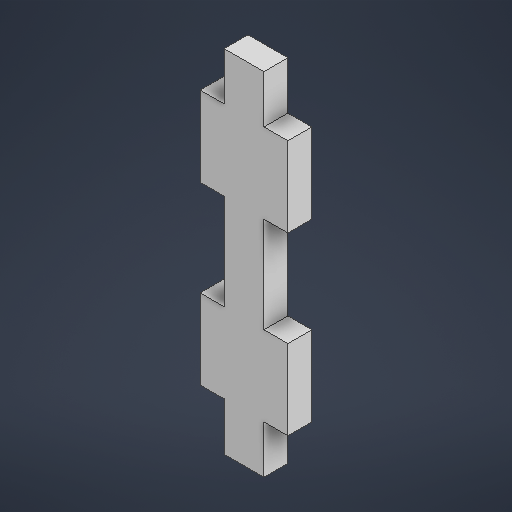
# Autodesk Inventor part: columna2
Saved by Autodesk Inventor 2026 (Build 300175000, 175)
## iProperties
Created: 2026-05-15
Part Number: columna2
Material: Generic
Document SubType Name: Modeling
Designer: juana
Density: 1 g/cm^3
Appearance: Default
Author: juana
Autodesk Inventor part; units mm, degrees
ref_plane "YZ Plane" through (0, 0, 0) normal (1, 0, 0) x (0, 1, 0)
ref_plane "XZ Plane" through (0, 0, 0) normal (0, 1, 0) x (-1, 0, 0)
ref_plane "XY Plane" through (0, 0, 0) normal (0, 0, 1) x (1, 0, 0)
sketch "Sketch1" plane through (0, 0, 0) normal (0, 0, 1) x (1, 0, 0)
  line L0 (0, 0) -> (5, 0)
  line L1 (5, 0) -> (5, 44)
  line L2 (5, 44) -> (0, 44)
  line L3 (0, 44) -> (0, 0)
  line L4 (5, 6) -> (8, 6)
  line L5 (8, 6) -> (8, 16)
  line L6 (8, 16) -> (5, 16)
  line L7 (5, 16) -> (5, 6)
  line L8 (5, 22) -> (0, 22) construction
  line L9 (2.5, 22) -> (2.5, 0) construction
  line L10 (0, 6) -> (-3, 6)
  line L11 (-3, 6) -> (-3, 16)
  line L12 (-3, 16) -> (0, 16)
  line L13 (5, 38) -> (8, 38)
  line L14 (8, 38) -> (8, 28)
  line L15 (8, 28) -> (5, 28)
  line L16 (-3, 28) -> (0, 28)
  line L17 (-3, 38) -> (-3, 28)
  line L18 (0, 38) -> (-3, 38)
  point P0 (6.5, 6)
  point P1 (-1.5, 6)
  point P2 (6.5, 38)
  point P3 (-1.5, 38)
  dimension "d0" = 5
  dimension "d1" = 44
  dimension "d2" = 3
  dimension "d3" = 6
  dimension "d4" = 10
  constraints: 38 end point, 15 symmetric about line, 5 midpoint, 4 parallel, 2 horizontal, 2 perpendicular, 1 horizontal alignment, 1 point on line, 1 vertical alignment
  measures "d0" distance of L1.end L2.end
  measures "d1" distance of L0.end L1.end
  measures "d2" distance of L5.end L6.end
  measures "d3" vertical distance of point (6.5, 6) L0.end
  measures "d4" distance of L4.end L5.end
extrude "Extrusion1" add sketch "Sketch1" along normal blind 3
body "Solid1"
